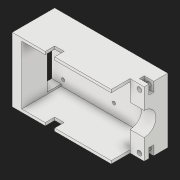
# Autodesk Inventor part: BP007
Saved by Autodesk Inventor 2017 SP1 (Build 210196100, 196)
## iProperties
Created: 2018-03-09
Part Number: BP007
Material: ABS Plastic
Document SubType Name: Modeling
Designer: Zach
Density: 1.06 g/cm^3
Appearance: CR White
Author: Zach
Autodesk Inventor part; units mm, degrees
ref_plane "YZ Plane" through (0, 0, 0) normal (1, 0, 0) x (0, 1, 0)
ref_plane "XZ Plane" through (0, 0, 0) normal (0, 1, 0) x (-1, 0, 0)
ref_plane "XY Plane" through (0, 0, 0) normal (0, 0, 1) x (1, 0, 0)
sketch "Sketch1" plane through (0, 0, 0) normal (0, 0, 1) x (1, 0, 0)
  line L0 (-27, 58.4) -> (108, 58.4)
  line L1 (108, 58.4) -> (108, -10)
  line L2 (108, -10) -> (-27, -10)
  line L3 (-27, -10) -> (-27, 58.4)
  circle A0 centre (82, 0) radius 1.7
  circle A1 centre (54, 5.5) radius 1.7
  circle A2 centre (54, 32.9) radius 1.7
  circle A3 centre (75.5, 48.4) radius 1.7
  circle A4 centre (1.5, 48.4) radius 1.7
  circle A5 centre (0, 0) radius 1.7
  dimension "d63" = 82
  dimension "d64" = 48.4
  dimension "d65" = 1.5
  dimension "d66" = 15.5
  dimension "d67" = 27.4
  dimension "d68" = 48.4
  dimension "d69" = 6.5
  dimension "d70" = 74
  dimension "d71" = 5.5
  dimension "d72" = 28
  dimension "d75" = 135
  dimension "d76" = 68.4
  dimension "d77" = 10
  dimension "d78" = 27
  dimension "d79" = 3.4
  dimension "d80" = 3.4
  dimension "d81" = 3.4
  dimension "d82" = 3.4
  dimension "d83" = 3.4
  dimension "d84" = 3.4
  constraints: 8 end point, 6 centre point, 2 parallel, 1 coincident, 1 horizontal, 1 perpendicular
  measures "d63" distance of A5.centre A0.centre
  measures "d64" vertical distance of A4.centre A5.centre
  measures "d65" horizontal distance of A5.centre A4.centre
  measures "d66" vertical distance of A2.centre A4.centre
  measures "d67" distance of A1.centre A2.centre
  measures "d68" vertical distance of A3.centre A0.centre
  measures "d69" horizontal distance of A0.centre A3.centre
  measures "d70" distance of A4.centre A3.centre
  measures "d71" vertical distance of A1.centre A0.centre
  measures "d72" horizontal distance of A0.centre A1.centre
  measures "d75" distance of L0.start L0.end
  measures "d76" distance of L0.end L1.end
  measures "d77" distance from line of L2 point (0, 0)
  measures "d78" distance from line of point (0, 0) L3
  measures "d79" diameter of A0
  measures "d80" diameter of A3
  measures "d81" diameter of A2
  measures "d82" diameter of A1
  measures "d83" diameter of A5
  measures "d84" diameter of A4
extrude "Extrusion1" add sketch "Sketch1" along normal blind 3
sketch "Sketch2" plane through (108, -10, 0) normal (1, 0, 0) x (0, 0, -1)
  circle A0 centre (-25, 34.2) radius 12.5 construction
  line L0 (-3, 0) -> (-3, 68.4) projected
  line L1 (0, 0) -> (-3, 0) projected
  line L2 (-3, 0) -> (-25, 0)
  line L3 (-25, 0) -> (-25, 68.4) construction
  line L4 (-25, 68.4) -> (-3, 68.4)
  line L5 (-25, 68.4) -> (-25, 46.7)
  line L6 (-25, 0) -> (-25, 21.7)
  arc A1 (-25, 21.7) -> (-25, 46.7) centre (-25, 34.2) ccw
  point P0 (0, 10)
  point P1 (-3, 34.2)
  point P2 (-3, 34.2)
  dimension "d23" = 25
  dimension "d24" = 22
  constraints: 10 end point, 4 point on circle, 3 midpoint, 2 centre point, 2 horizontal, 2 point on line, 1 concentric, 1 horizontal alignment, 1 perpendicular
  measures "d23" diameter of A0
  measures "d24" distance from line of L0 A0.centre
extrude "Extrusion2" add sketch "Sketch2" against normal blind 15
sketch "Sketch3" plane through (108, -10, 25) normal (0, 0, 1) x (1, 0, 0)
  circle A0 centre (-5, 5) radius 2.5
  line L0 (0, 0) -> (-15, 0) projected
  line L1 (0, 21.7) -> (0, 0) projected
  point P0 (-108, 10)
  dimension "d28" = 5
  dimension "d29" = 5
  dimension "d30" = 5
  constraints: 1 centre point
  measures "d28" diameter of A0
  measures "d29" distance from line of L0 A0.centre
  measures "d30" distance from line of L1 A0.centre
extrude "Extrusion3" cut sketch "Sketch3" against normal through all
sketch "Sketch4" plane through (0, 0, 3) normal (0, 0, 1) x (1, 0, 0)
  line L0 (-27, 58.4) -> (108, 58.4) projected
  line L1 (-27, 58.4) -> (-2, 58.4)
  line L2 (-2, 58.4) -> (-2, -10)
  line L3 (-2, -10) -> (-27, -10)
  line L4 (-27, -10) -> (-27, 58.4)
  point P0 (0, 0)
  point P1 (93, -10)
  dimension "d33" = 25
  constraints: 8 end point, 2 parallel, 1 horizontal, 1 horizontal alignment, 1 perpendicular
  measures "d33" distance between parallel lines of L4 L2
extrude "Extrusion4" add sketch "Sketch4" along normal blind 42
sketch "Sketch5" plane through (-2, -10, 3) normal (1, 0, 0) x (0, 0, -1)
  line L0 (0, 68.4) -> (0, 0) projected
  line L1 (0, 0) -> (0, 68.4) projected
  line L2 (0, 5) -> (-15, 5)
  line L3 (-15, 5) -> (-15, 63.4)
  line L4 (-15, 63.4) -> (0, 63.4)
  line L5 (0, 63.4) -> (0, 5)
  line L6 (3, 68.4) -> (-42, 68.4) projected
  point P0 (3, 10)
  point P1 (0, 8.3)
  point P2 (0, 11.7)
  point P3 (0, 23.8)
  point P4 (0, 27.2)
  point P5 (0, 51.2)
  point P6 (0, 54.6)
  point P7 (0, 56.7)
  point P8 (0, 60.1)
  point P9 (0, 56.7)
  point P10 (0, 60.1)
  point P11 (0, 8.3)
  point P12 (0, 11.7)
  dimension "d36" = 5
  dimension "d37" = 5
  dimension "d38" = 15
  constraints: 8 end point, 2 parallel, 1 horizontal, 1 perpendicular, 1 point on line
  measures "d36" distance from line of L0.end L2
  measures "d37" distance from line of L6 L4.end
  measures "d38" distance between parallel lines of L5 L3
extrude "Extrusion5" cut sketch "Sketch5" against normal through all
sketch "Sketch6" plane through (0, 0, 3) normal (0, 0, 1) x (1, 0, 0)
  line L0 (-2, -10) -> (93, -10) projected
  line L1 (93, -10) -> (93, 58.4) projected
  line L2 (-2, -10) -> (93, -10)
  line L3 (93, -10) -> (93, -7)
  line L4 (93, -7) -> (-2, -7)
  line L5 (-2, -7) -> (-2, -10)
  line L6 (93, 58.4) -> (-2, 58.4) projected
  line L7 (-2, 58.4) -> (93, 58.4)
  line L8 (93, 58.4) -> (93, 55.4)
  line L9 (93, 55.4) -> (-2, 55.4)
  line L10 (-2, 55.4) -> (-2, 58.4)
  point P0 (0, 0)
  dimension "d41" = 3
  dimension "d42" = 3
  constraints: 16 end point, 4 parallel, 2 horizontal, 2 perpendicular, 2 point on line
  measures "d41" distance between parallel lines of L6 L9
  measures "d42" distance between parallel lines of L0 L4
extrude "Extrusion6" add sketch "Sketch6" along normal blind 42
sketch "Sketch7" plane through (108, 36.7, 25) normal (0, 0, 1) x (1, 0, 0)
  circle A0 centre (-5, 16.7) radius 2.5
  line L0 (0, 21.7) -> (-15, 21.7) projected
  point P0 (-108, -36.7)
  dimension "d45" = 5
  dimension "d46" = 5
  dimension "d47" = 5
  constraints: 1 centre point
  measures "d45" diameter of A0
  measures "d46" distance from line of L0 A0.centre
  measures "d47" horizontal distance of L0.start A0.centre
extrude "Extrusion7" cut sketch "Sketch7" against normal through all
sketch "Sketch9" plane through (-2, 55.4, 3) normal (0, -1, 0) x (1, 0, 0)
  line L0 (0, 42) -> (95, 42) projected
  line L1 (25, 42) -> (35, 42)
  line L2 (35, 42) -> (35, 32)
  line L3 (35, 32) -> (25, 32)
  line L4 (25, 32) -> (25, 42)
  point P0 (2, -3)
  dimension "d50" = 25
  dimension "d51" = 10
  dimension "d52" = 10
  constraints: 8 end point, 2 parallel, 1 horizontal, 1 perpendicular, 1 point on line
  measures "d50" distance from line of L0.start L4
  measures "d51" distance of L1.end L2.end
  measures "d52" distance between parallel lines of L2 L4
extrude "Extrusion8" cut sketch "Sketch9" along normal through all both and the other way through all
sketch "Sketch10" plane through (108, -10, 0) normal (1, 0, 0) x (0, 0, -1)
  line L0 (0, 7.5) -> (0, 2.5) projected
  line L1 (-25, 2.5) -> (-25, 7.5) projected
  line L2 (0, 65.9) -> (0, 60.9) projected
  line L3 (-25, 60.9) -> (-25, 65.9) projected
  line L4 (0, 0) -> (-45, 0) projected
  line L5 (-20, 0) -> (-15, 0)
  line L6 (-15, 0) -> (-15, 10)
  line L7 (-15, 10) -> (-20, 10)
  line L8 (-20, 10) -> (-20, 0)
  line L9 (0, 68.4) -> (-45, 68.4) projected
  line L10 (-20, 68.4) -> (-15, 68.4)
  line L11 (-15, 68.4) -> (-15, 58.4)
  line L12 (-15, 58.4) -> (-20, 58.4)
  line L13 (-20, 58.4) -> (-20, 68.4)
  point P0 (0, 10)
  dimension "d55" = 5
  dimension "d56" = 10
  dimension "d57" = 5
  dimension "d58" = 10
  constraints: 16 end point, 4 parallel, 2 horizontal, 2 perpendicular, 2 point on line, 2 vertical alignment
  measures "d55" distance of L7.end L6.end
  measures "d56" distance of L6.end L5.end
  measures "d57" distance between parallel lines of L1 L8
  measures "d58" distance of L10.end L11.end
extrude "Extrusion9" cut sketch "Sketch10" against normal blind 10
sketch "Sketch12" plane through (0, 0, 45) normal (0, 0, 1) x (1, 0, 0)
  line L0 (23, 58.4) -> (-27, 58.4) projected
  line L1 (-27, -10) -> (23, -10) projected
  line L2 (-27, 58.4) -> (-12, 58.4)
  line L3 (-12, 58.4) -> (-12, -10)
  line L4 (-12, -10) -> (-27, -10)
  line L5 (-27, -10) -> (-27, 58.4)
  line L6 (-2, -7) -> (-2, 55.4) projected
  point P0 (0, 0)
  dimension "d85" = 10
  constraints: 8 end point, 2 parallel, 1 horizontal, 1 perpendicular, 1 point on line
  measures "d85" distance between parallel lines of L6 L3
extrude "Extrusion10" cut sketch "Sketch12" against normal through all
body "Solid1"
